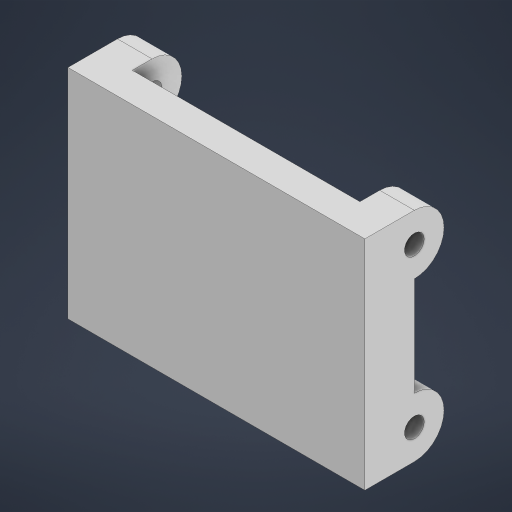
# Autodesk Inventor part: Motor_Base
Saved by Autodesk Inventor 2024 (Build 280153000, 153)
## iProperties
Created: 2024-06-01
Part Number: Motor_Base
Material: Generic
Document SubType Name: Modeling
Designer: Hemant
Density: 1 g/cm^3
Appearance: Default
Author: Hemant
Autodesk Inventor part; units mm, degrees
ref_plane "YZ Plane" through (0, 0, 0) normal (1, 0, 0) x (0, 1, 0)
ref_plane "XZ Plane" through (0, 0, 0) normal (0, 1, 0) x (-1, 0, 0)
ref_plane "XY Plane" through (0, 0, 0) normal (0, 0, 1) x (1, 0, 0)
sketch "Sketch1" plane through (0, 0, 0) normal (0, 0, 1) x (1, 0, 0)
  line L0 (-11.5, 11) -> (11.5, 11)
  line L1 (11.5, 11) -> (11.5, -11)
  line L2 (11.5, -11) -> (-11.5, -11)
  line L3 (-11.5, -11) -> (-11.5, 11)
  line L4 (-11.5, 11) -> (11.5, -11) construction
  line L5 (11.5, 11) -> (-11.5, -11) construction
  point P0 (0, 0)
  dimension "d0" = 23
  dimension "d1" = 22
  constraints: 12 end point, 2 midpoint, 2 parallel, 1 horizontal, 1 perpendicular
  measures "d0" distance of L1.end L2.end
  measures "d1" distance of L0.end L1.end
extrude "Extrusion1" add sketch "Sketch1" along normal blind 3
sketch "Sketch2" plane through (0, 0, 3) normal (0, 0, 1) x (1, 0, 0)
  line L0 (11.5, 11) -> (-11.5, 11) projected
  line L1 (-11.5, 11) -> (-15, 11)
  line L2 (-15, 11) -> (-15, -11)
  line L3 (-15, -11) -> (-11.5, -11)
  line L4 (-11.5, -11) -> (-11.5, 11)
  line L5 (-11.5, -11) -> (11.5, -11) projected
  line L6 (11.5, -11) -> (15, -11)
  line L7 (15, -11) -> (15, 11)
  line L8 (15, 11) -> (11.5, 11)
  line L9 (11.5, 11) -> (11.5, -11)
  point P0 (0, 0)
  dimension "d4" = 3.5
  dimension "d5" = 3.5
  constraints: 16 end point, 4 parallel, 2 horizontal, 2 perpendicular, 1 point on line
  measures "d4" distance of L3.end L2.end
  measures "d5" distance of L8.end L7.end
extrude "Extrusion2" add sketch "Sketch2" against normal blind 8.5 contours L8 L7 L6 L9 | L4 L3 L2 L1
sketch "Sketch3" plane through (15, -11, 3) normal (1, 0, 0) x (0, 0, -1)
  line L0 (0, 0) -> (0, 22) construction
  line L1 (0, 22) -> (8.5, 22) construction
  line L2 (8.5, 22) -> (8.5, 0) construction
  line L3 (8.5, 0) -> (0, 0) construction
  circle A0 centre (5, 19) radius 1
  circle A1 centre (5, 3) radius 1
  line L4 (3, 22) -> (3, 0) construction
  arc A2 (5, 16) -> (5, 22) centre (5, 19) ccw
  line L5 (5, 22) -> (5, 0) construction
  arc A3 (5, 0) -> (5, 6) centre (5, 3) ccw
  line L6 (5, 16) -> (5, 6)
  line L7 (3, 22) -> (8.5, 22) projected
  line L8 (5, 0) -> (8.5, 0)
  line L9 (8.5, 0) -> (8.5, 22)
  line L10 (8.5, 22) -> (5, 22)
  point P0 (3, 11)
  point P1 (3, 11)
  dimension "d8" = 2
  dimension "d9" = 2
  dimension "d10" = 16
  dimension "d11" = 2
  dimension "d12" = 8
  constraints: 10 end point, 4 centre point, 4 point on circle, 4 point on line, 2 coincident, 2 collinear, 1 horizontal, 1 midpoint, 1 perpendicular, 1 tangent, 1 vertical alignment
  measures "d8" diameter of A0
  measures "d9" diameter of A1
  measures "d10" distance of A1.centre A0.centre
  measures "d11" distance from line of L4 A0.centre
  measures "d12" vertical distance of A0.centre point (3, 11)
extrude "Extrusion3" cut sketch "Sketch3" against normal through all
sketch "Sketch4" plane through (15, -11, 3) normal (1, 0, 0) x (0, 0, -1)
  line L0 (0, 0) -> (0, 22) projected
  line L1 (0, 21.5) -> (5, 21.5)
  line L2 (5, 21.5) -> (5, 23.5)
  line L3 (5, 23.5) -> (0, 23.5)
  line L4 (0, 23.5) -> (0, 21.5)
  line L5 (0, 22) -> (5, 22) projected
  line L6 (0, 0.5) -> (5, 0.5)
  line L7 (5, 0.5) -> (5, -1.5)
  line L8 (5, -1.5) -> (0, -1.5)
  line L9 (0, -1.5) -> (0, 0.5)
  line L10 (0, 0) -> (5, 0) projected
  dimension "d21" = 5
  dimension "d22" = 2
  dimension "d23" = 0.5
  dimension "d24" = 5
  dimension "d25" = 2
  dimension "d26" = 0.5
  constraints: 16 end point, 4 parallel, 2 horizontal, 2 perpendicular, 2 point on line
  measures "d21" distance of L3.end L2.end
  measures "d22" distance of L2.end L1.end
  measures "d23" distance between parallel lines of L1 L5
  measures "d24" distance of L7.end L8.end
  measures "d25" distance of L6.end L7.end
  measures "d26" distance between parallel lines of L10 L6
extrude "Extrusion4" [suppressed]
equation "\"d12\" = 0.5 * d10"
body "Solid1"
